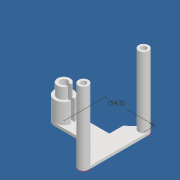
# Autodesk Inventor part: HolderShaft
Saved by Autodesk Inventor 2020 (Build 240168000, 168)
## iProperties
Created: 2019-12-14
Part Number: HolderShaft
Material: Generic
Document SubType Name: Modeling
Designer: Jack
Density: 1 g/cm^3
Appearance: Default
Author: Jack
Autodesk Inventor part; units mm, degrees
ref_plane "YZ Plane" through (0, 0, 0) normal (1, 0, 0) x (0, 1, 0)
ref_plane "XZ Plane" through (0, 0, 0) normal (0, 1, 0) x (-1, 0, 0)
ref_plane "XY Plane" through (0, 0, 0) normal (0, 0, 1) x (1, 0, 0)
sketch "Sketch1" plane through (0, 0, 0) normal (0, 1, 0) x (-1, 0, 0)
  circle A0 centre (0, 0) radius 7
  circle A1 centre (0, 0) radius 4
  dimension "d0" = 14
  dimension "d1" = 8
  constraints: 2 centre point, 2 coincident
  measures "d0" diameter of A0
  measures "d1" diameter of A1
extrude "Extrusion1" add sketch "Sketch1" along normal blind 12
sketch "Sketch5" plane through (0, 0, 0) normal (0, -1, 0) x (1, 0, 0)
  circle A0 centre (0, 0) radius 10
  dimension "d17" = 20
  constraints: 1 centre point, 1 coincident
  measures "d17" diameter of A0
extrude "Extrusion3" add sketch "Sketch5" along normal blind 25
hole "Hole2" at (0, 0, 0) direction (0, -1, 0) diameter 8 depth 22
sketch "Sketch6" plane through (0, 0, 0) normal (1, 0, 0) x (0, 1, 0)
  line L0 (-25, 10) -> (-25, -10) projected
  line L1 (0, 10) -> (-25, 10) projected
  line L2 (-25, -10) -> (-22, -10)
  line L3 (-22, -10) -> (-22, 10)
  line L4 (-22, 10) -> (-25, 10)
  line L5 (-25, 10) -> (-25, -10)
  point P0 (0, 0)
  dimension "d29" = 3
  constraints: 8 end point, 2 parallel, 1 horizontal, 1 perpendicular, 1 point on line
  measures "d29" distance of L0.end L2.end
extrude "Extrusion4" add sketch "Sketch6" along normal blind 60
sketch "Sketch7" plane through (0, 0, 0) normal (0, 0, 1) x (1, 0, 0)
  line L0 (12.4966, 12) -> (0.0574, 12)
  line L1 (0.0574, 12) -> (0.0574, -22)
  line L2 (0.0574, -22) -> (12.4966, -22)
  line L3 (12.4966, -22) -> (12.4966, 12)
  line L4 (7, 12) -> (-7, 12) projected
  line L5 (0, -22) -> (60, -22) projected
  line L6 (8.0699, 12) -> (-5.9211, 12) projected
  point P0 (0, 0)
  constraints: 8 end point, 2 collinear, 2 parallel, 1 perpendicular
extrude "Extrusion5" cut sketch "Sketch7" along normal mid plane 4
sketch "Sketch8" plane through (0, 0, 0) normal (0, 0, 1) x (1, 0, 0)
  line L0 (0, -22) -> (60, -22) projected
  line L1 (0, -25) -> (60, -25) projected
  line L2 (60, -22) -> (40, -22)
  line L3 (40, -22) -> (40, -25)
  line L4 (40, -25) -> (60, -25)
  line L5 (60, -25) -> (60, -22)
  point P0 (0, 0)
  dimension "d43" = 20
  constraints: 8 end point, 2 parallel, 1 horizontal, 1 perpendicular, 1 point on line
  measures "d43" distance of L4.end L3.end
extrude "Extrusion6" add sketch "Sketch8" along normal mid plane 50
sketch "Sketch9" plane through (0, -25, 0) normal (0, -1, 0) x (1, 0, 0)
  circle A0 centre (54.5, -33) radius 5.5
  line L0 (60, -25) -> (60, 25) projected
  line L1 (60, -25) -> (40, -25) projected
  point P0 (0, 0)
  dimension "d48" = 5.5
  dimension "d49" = 11
  dimension "d66" = 8
  constraints: 1 centre point, 1 coincident
  measures "d48" distance from line of L0 A0.centre
  measures "d49" diameter of A0
  measures "d66" distance from line of L1 A0.centre
extrude "Extrusion7" add sketch "Sketch9" against normal blind 80
sketch "Sketch11" plane through (54.5, 55, -33) normal (0, 1, 0) x (1, 0, 0)
  point P0 (-54.5, -33)
  point P1 (0, 0)
hole "Hole3" at (54.5, 55, -33) direction (0, -1, 0) diameter 6 depth 77
sketch "Sketch12" plane through (54.5, -25, -33) normal (0, -1, 0) x (1, 0, 0)
  line L0 (-14.5, 8) -> (5.5, 8) projected
  line L1 (5.5, 8) -> (5.5, 0)
  circle A0 centre (0, 0) radius 5.5 projected
  line L2 (5.5, 8) -> (-14.5, 8)
  line L3 (-14.5, 8) -> (-5.5, 0)
  line L4 (-5.5, 0) -> (5.5, 0)
  line L5 (-14.5, 58) -> (5.5, 58) projected
  line L6 (5.5, 58) -> (5.5, 66)
  line L7 (5.5, 66) -> (-5.5, 66)
  line L8 (-5.5, 66) -> (-14.5, 58)
  line L9 (-14.5, 58) -> (5.5, 58)
  point P0 (-54.5, 33)
  dimension "d61" = 8
  dimension "d62" = 8
  dimension "d63" = 11
  dimension "d64" = 20
  dimension "d65" = 11
  constraints: 16 end point, 2 collinear, 2 point on circle, 2 vertical, 1 horizontal, 1 perpendicular
  measures "d61" distance of L5.end L6.end
  measures "d62" distance of L0.end L1.end
  measures "d63" distance of L3.end L1.end
  measures "d64" distance of L0.start L0.end
  measures "d65" distance of L6.end L7.end
extrude "Extrusion8" add sketch "Sketch12" against normal blind 3 contours L0 L1 A0 L3 | A0 L4 | L8 L7 L6 L5 picked at (-1.8333, 1.704)
mirror "Mirror1" about plane through (0, 0, 0) normal (0, 0, 1) of "Extrusion7"
sketch "Sketch13" plane through (54.5, 55, 33) normal (0, 1, 0) x (1, 0, 0)
  point P0 (-54.5, 33)
  point P1 (0, 0)
hole "Hole4" at (54.5, 55, 33) direction (0, -1, 0) diameter 6 depth 77
sketch "Sketch15" plane through (0, -25, 0) normal (0, -1, 0) x (1, 0, 0)
  circle A0 centre (54.5, -33) radius 5.5 projected
  circle A1 centre (54.5, 33) radius 5.5 projected
  arc A2 (3.4641, 2) -> (3.4641, -2) centre (0, 0) ccw projected
  arc A3 (6.7082, 2) -> (6.7082, -2) centre (0, 0) ccw projected
  circle A4 centre (54.5, -33) radius 3 projected
  dimension "d74" = 54.5
  dimension "d75" = 7
  dimension "d77" = 4
  dimension "d78" = 6
  dimension "d80" = 33
  dimension "d82" = 11
  measures "d74" horizontal distance of point (0, 0) A0.centre
  measures "d75" radius of A3
  measures "d77" radius of A2
  measures "d78" diameter of A4
  measures "d80" vertical distance of A0.centre point (0, 0)
  measures "d82" diameter of A1
sketch "Sketch16" plane through (0, 0, 2) normal (0, 0, -1) x (-1, 0, 0)
  line L0 (7, 12) -> (-6.7082, 12) projected
  line L1 (0, -22) -> (-40, -22) projected
  line L2 (-49, -22) -> (-40, -22) projected
  line L3 (-49, 55) -> (-60, 55) projected
  point P0 (0, 0)
  dimension "d79" = 34
  dimension "d81" = 77
  measures "d79" distance between parallel lines of L1 L0
  measures "d81" distance between parallel lines of L2 L3
equation "\"d61\" = d62"
equation "\"d65\" = d63"
body "Solid1"
